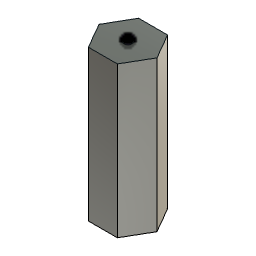
_pcb-post.2ef064a2-71a8-4e5f-af67-261210c2e70e (Autodesk Fusion 360 design; units mm, degrees)
Autodesk Fusion 360 part; units mm, degrees
sketch "Sketch1" plane through (0, 0, 0) normal (0, 0, 1) x (1, 0, 0)
  line L0 (-5.7735, 10) -> (-11.547, 0)
  line L1 (-11.547, 0) -> (-5.7735, -10)
  line L2 (-5.7735, -10) -> (5.7735, -10)
  line L3 (5.7735, -10) -> (11.547, 0)
  line L4 (11.547, 0) -> (5.7735, 10)
  line L5 (5.7735, 10) -> (-5.7735, 10)
  dimension "d1" = 10
  measures "d1" distance of origin L5
extrude "Extrude1" add sketch "Sketch1" along normal blind 60
sketch "Sketch2" plane through (0, 0, 60) normal (0, 0, 1) x (-1, 0, 0)
  line L0 (-5.7735, -10) -> (5.7735, -10)
  line L1 (5.7735, -10) -> (11.547, 0)
  line L2 (11.547, 0) -> (5.7735, 10)
  line L3 (5.7735, 10) -> (-5.7735, 10)
  line L4 (-5.7735, 10) -> (-11.547, 0)
  line L5 (-11.547, 0) -> (-5.7735, -10)
  circle A0 centre (0, 0) radius 1.6
  dimension "d4" = 3.2
  constraint coincident A0.centre origin
  measures "d4" diameter of A0
extrude "Extrude3" cut sketch "Sketch2" against normal blind 10 contours A0
sketch "Sketch4" plane through (0, 0, 0) normal (0, 0, -1) x (1, 0, 0)
  line L0 (-5.7735, -10) -> (5.7735, -10)
  line L1 (5.7735, -10) -> (11.547, 0)
  line L2 (11.547, 0) -> (5.7735, 10)
  line L3 (5.7735, 10) -> (-5.7735, 10)
  line L4 (-5.7735, 10) -> (-11.547, 0)
  line L5 (-11.547, 0) -> (-5.7735, -10)
  circle A0 centre (0, 0) radius 2.625
  dimension "d9" = 5.25
  constraint coincident A0.centre origin
  measures "d9" diameter of A0
extrude "Extrude4" cut sketch "Sketch4" against normal blind 10 contours A0
